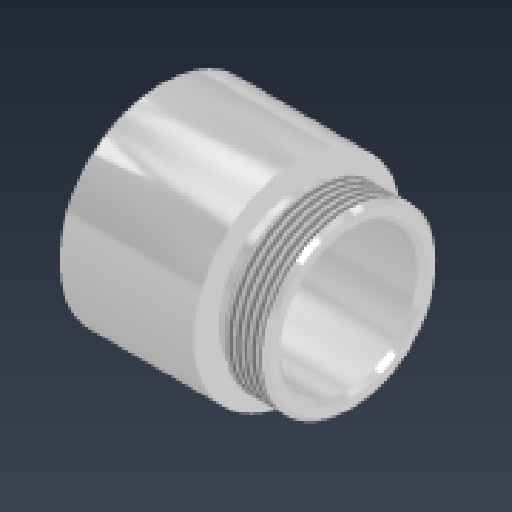
# Autodesk Inventor part: PommelPart
Saved by Autodesk Inventor 2025.1 (Build 291241000, 241)
## iProperties
Created: 2024-08-20
Part Number: PommelPart
Material: Aluminum 6061
Document SubType Name: Modeling
Designer: Michael
Density: 2.7 g/cm^3
Appearance: Aluminum - Flat
Mass: 55.3052 g
Surface Area: 90.0919 cm^2
Volume: 20.4834 cm^3
Author: Michael
Autodesk Inventor part; units mm, degrees
ref_plane "YZ Plane" through (0, 0, 0) normal (1, 0, 0) x (0, 1, 0)
ref_plane "XZ Plane" through (0, 0, 0) normal (0, 1, 0) x (-1, 0, 0)
ref_plane "XY Plane" through (0, 0, 0) normal (0, 0, 1) x (1, 0, 0)
sketch "Sketch1" plane through (0, 0, 0) normal (0, 0, 1) x (1, 0, 0)
  line L0 (-30.2941, 0) -> (30.2941, 0)
  line L1 (-14.605, 12.7) -> (14.605, 12.7)
  line L2 (14.605, 12.7) -> (14.605, 16.002)
  line L3 (14.605, 16.002) -> (6.985, 16.002)
  line L4 (6.985, 16.002) -> (6.985, 14.478)
  line L5 (6.985, 14.478) -> (4.445, 14.478)
  line L6 (4.445, 14.478) -> (4.445, 19.05)
  line L7 (4.445, 19.05) -> (-20.955, 19.05)
  line L8 (-20.955, 19.05) -> (-20.955, 9.525)
  line L9 (-20.955, 9.525) -> (-14.605, 9.525)
  line L10 (-14.605, 9.525) -> (-14.605, 12.7)
  point P0 (0, 0)
  point P1 (0, 0)
  point P2 (0, 12.7)
  dimension "d0" = 25.4
  dimension "d2" = 19.05
  dimension "d3" = 6.35
  dimension "d4" = 38.1
  dimension "d6" = 19.05
  dimension "d7" = 32.004
  dimension "d8" = 1.524
  dimension "d16" = 10.16
  dimension "d17" = 2.54
  constraints: 22 end point, 8 perpendicular, 2 horizontal, 2 midpoint, 1 coincident, 1 vertical, 1 vertical alignment
  measures "d0" diameter of L1 L0
  measures "d2" distance between parallel lines of L10 L6
  measures "d3" distance between parallel lines of L8 L10
  measures "d4" diameter of L7 L0
  measures "d6" diameter of L9 L0
  measures "d7" diameter of L3 L0
  measures "d8" distance between parallel lines of L3 L5
  measures "d16" distance between parallel lines of L2 L6
  measures "d17" distance between parallel lines of L6 L4
revolve "Revolution1" add sketch "Sketch1" angle 360 about axis through (-30.2941, 0, 0) along (1, 0, 0)
thread "Thread1" size "1 1/4-18 UNEF" class "2A" standard "ANSI Unified Screw Threads" full length
chamfer "Chamfer1" distance 0.7937 angle 45 5 edges at (14.605, -16.002, 0) (14.605, -12.7, 0) (-14.605, -9.525, 0) (-20.955, -9.525, 0) (-20.955, -19.05, 0)
body "Solid1"
